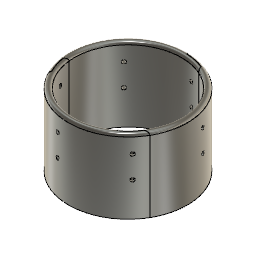
modified_drum (1) (Autodesk Fusion 360 design; units mm, degrees)
Autodesk Fusion 360 part; units mm, degrees
sketch "Sketch1" plane through (0, 0, 0) normal (0, 0, 1) x (1, 0, 0)
  arc A0 (96.5614, 31.5984) -> (-0.2128, 101.5998) centre (0, 0) ccw
  line L0 (0, 0) -> (96.5614, 31.5984) construction
  line L1 (0, 0) -> (-0.2128, 101.5998) construction
  arc A1 (91.8093, 30.0434) -> (-0.2023, 96.5998) centre (0, 0) ccw
  arc A2 (87.0573, 28.4884) -> (-0.1918, 91.5998) centre (0, 0) ccw
  line L2 (-0.2128, 101.5998) -> (-0.1918, 91.5998)
  line L3 (96.5614, 31.5984) -> (87.0573, 28.4884)
  arc A3 (41.13, 92.9026) -> (-0.2128, 101.5998) centre (0, 0) ccw
  line L4 (0, 0) -> (41.13, 92.9026) construction
  line L5 (0, 0) -> (-0.2128, 101.5998) construction
  line L6 (41.13, 92.9026) -> (37.0817, 83.7586)
  line L7 (-0.2128, 101.5998) -> (4.9346, 96.4739)
  line L8 (-0.2128, 101.5998) -> (-129.4294, 101.5998) construction
  line L9 (37.0817, 83.7586) -> (34.5966, 90.1922)
  arc A4 (59.891, -82.0709) -> (96.5614, 31.5984) centre (0, 0) ccw
  arc A5 (53.9962, -73.993) -> (87.0573, 28.4884) centre (0, 0) ccw
  line L10 (0, 0) -> (59.891, -82.0709) construction
  line L11 (0, 0) -> (59.891, -82.0709) construction
  line L12 (0, 0) -> (88.0944, -50.6156) construction
  line L13 (59.891, -82.0709) -> (61.0124, -74.8936)
  arc A6 (56.9436, -78.032) -> (91.8093, 30.0434) centre (0, 0) ccw
  line L14 (59.891, -82.0709) -> (53.9962, -73.993)
  line L15 (0, 0) -> (96.5614, 31.5984) construction
  line L16 (79.4237, -45.6338) -> (81.2227, -52.2919)
  line L17 (59.891, -82.0709) -> (-44.3284, -158.4597) construction
  line L18 (88.0944, -50.6156) -> (79.4237, -45.6338)
  line L19 (96.5614, 31.5984) -> (87.0573, 28.4884)
  arc A7 (59.891, -82.0709) -> (88.0944, -50.6156) centre (0, 0) ccw
  line L20 (88.0944, -50.6156) -> (81.0815, -52.5104)
  line L21 (53.9962, -73.993) -> (60.8104, -75.0577)
  dimension "d1" = 101.6
  dimension "d2" = 72
  dimension "d5" = 24
  dimension "d7" = 45
  dimension "d8" = 45
  dimension "d9" = 45
  dimension "d12" = 45
  constraint coincident A0.centre L0.start
  constraint parallel L1 L2
  constraint parallel L0 L3
  constraint coincident A1.start L3
  constraint coincident A1.end L2
  constraint coincident L4 L6.end
  constraint coincident A2 L6.end
  constraint horizontal L8
  constraint coincident A1 L7.end
  constraint coincident A1 L9.end
  constraint symmetric A0.centre L3 L0.start
  constraint symmetric A0.start L3 L0.end
  constraint symmetric A0.end L3 A4.start
  constraint symmetric A0 L3 A4
  constraint symmetric A1.start L3 A6.end
  constraint symmetric A1.end L3 A6.start
  constraint symmetric A1 L3 A6
  constraint symmetric A2.start L3 A5.end
  constraint symmetric A2.end L3 A5.start
  constraint symmetric A2 L3 A5
  constraint symmetric L3 A3.start L12.end
  constraint symmetric L3 A3 A7
  constraint symmetric L3 L6.end L16.start
  constraint symmetric L3 L7.end L13.end
  constraint symmetric L3 L8.end L17.end
  constraint symmetric L3 L9.end L16.end
  constraint coincident A6 L20.end
  constraint coincident A6 L21.end
  measures "d1" radius of A0
  measures "d2" angle of L0 L1
  measures "d5" angle of L4 L5
  measures "d7" angle of L6 L9
  measures "d8" angle of L18 L20
  measures "d9" angle of L14 L21
  measures "d12" angle of L2 L7
extrude "Extrude1" add sketch "Sketch1" along normal blind 127 contours A0 A1 L3 L6 L19 | L3 A4 A6 L18 L19 | A0 A1 A3 L6 L7 | A1 A2 L3 L6 L19 | L3 A5 A6 L18 L19 | A6 L18 L20 | A1 L6 L9 | A6 L16 L18 | A5 A6 L16 L21 makes body 1
fillet "Fillet1" radius 5 2 edges at (91.078, 9.7656, 127) (87.8816, 50.9842, 127) on bodies 1
ref_plane "WorkPlane1" through (96.5614, 31.5984, 0) normal (0.950407, 0.311008, 0) x (-0.311008, 0.950407, 0)
sketch "Sketch2" plane through (96.5614, 31.5984, 0) normal (0.950407, 0.311008, 0) x (-0.311008, 0.950407, 0)
  line L0 (0, 122) -> (0, 96.6)
  line L1 (0, 96.6) -> (0, 58.5)
  line L2 (96.6273, 122) -> (-75.5035, 122)
  dimension "d24" = 25.4
  dimension "d25" = 38.1
  constraint vertical L0
  constraint parallel L0 L1
  constraint coincident L0.start L2
  measures "d24" distance of L0.start L0.end
  measures "d25" distance of L0.end L1.end
hole "Hole1" at (96.5614, 31.5984, 96.6) at (96.5614, 31.5984, 58.5) direction (-0.950407, -0.311008, 0) diameter 6.35 depth 12.7 tip angle 118 bodies 1
pattern_circular "C-Pattern2" count 6 over 360 about axis through (0, 0, 122) along (0, 0, 1) of "Hole1"
pattern_circular "C-Pattern3" count 3 over 360 about axis through (0, 0, 122) along (0, 0, 1) of bodies 1 makes body 2 at (5.145, 91.4554, 60.2494) makes body 3 at (-81.7748, -41.2728, 60.0962)
equation "d1 = ShellDiam / 2"
equation "d2 = PieceSize * LapSize + PieceSize"
equation "d3 = -HalfShellThick"
equation "d4 = -ShellThick"
equation "d5 = PieceSize * ( LapSize * 2 )"
equation "d10 = ShellHeight"
equation "NumSegments = 3"
equation "ShellThick = 10 mm"
equation "ShellHeight = 5 in"
equation "ShellDiam = 8 in"
equation "LapSize = LapSizePercent / 100"
equation "PieceSize = ( 180 / NumSegments ) * 1 deg"
equation "d22 = HalfShellThick"
equation "d24 = LugTopDist"
equation "d25 = LugSpacing"
equation "d27 = LugHoleDiam"
equation "d29 = NumSegments * 2"
equation "d31 = NumSegments"
equation "LugTopDist = 1 in"
equation "LugSpacing = 1.5 in"
equation "LapSizePercent = 20"
equation "HalfShellThick = ShellThick / 2"
equation "LugHoleDiam = 0.25 in"
